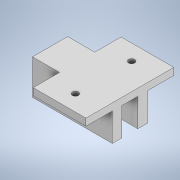
# Autodesk Inventor part: pulleysupport
Saved by Autodesk Inventor 2020.2 (Build 242310000, 310)
## iProperties
Created: 2020-08-06
Part Number: pulleysupport
Material: Generic
Document SubType Name: Modeling
Designer: JK
Density: 1 g/cm^3
Appearance: Default
Author: JK
Autodesk Inventor part; units mm, degrees
ref_plane "YZ Plane" through (0, 0, 0) normal (1, 0, 0) x (0, 1, 0)
ref_plane "XZ Plane" through (0, 0, 0) normal (0, 1, 0) x (-1, 0, 0)
ref_plane "XY Plane" through (0, 0, 0) normal (0, 0, 1) x (1, 0, 0)
sketch "Sketch1" plane through (0, 0, 0) normal (0, 1, 0) x (-1, 0, 0)
  line L0 (-15, 25) -> (15, 25)
  line L1 (15, 25) -> (15, -25)
  line L2 (15, -25) -> (-15, -25)
  line L3 (-15, -25) -> (-15, 25)
  line L4 (-15, 25) -> (15, -25) construction
  line L5 (15, 25) -> (-15, -25) construction
  circle A0 centre (0, 16) radius 1.75
  circle A1 centre (0, -16) radius 1.75
  point P0 (0, 0)
  dimension "d0" = 3.5
  dimension "d1" = 30
  dimension "d2" = 50
  dimension "d3" = 16
  dimension "d4" = 16
  constraints: 12 end point, 2 centre point, 2 midpoint, 2 parallel, 1 equal radius, 1 horizontal, 1 perpendicular
  measures "d0" diameter of A0
  measures "d1" distance of L0.start L0.end
  measures "d2" distance of L0.end L1.end
  measures "d3" distance of A0.centre point (0, 0)
  measures "d4" distance of A1.centre point (0, 0)
extrude "Extrusion1" add sketch "Sketch1" along normal blind 4
sketch "Sketch2" plane through (0, 4, 0) normal (0, 1, 0) x (1, 0, 0)
  line L0 (15, -25) -> (15, 25) projected
  line L1 (15, -10) -> (-30.3844, -10)
  line L2 (-30.3844, -10) -> (-30.3844, 10)
  line L3 (-30.3844, 10) -> (15, 10)
  line L4 (15, 10) -> (15, -10)
  line L5 (-15, -25) -> (15, -25) projected
  point P0 (0, 0)
  point P1 (15, 10)
  dimension "d9" = 20
  dimension "d11" = 10
  constraints: 8 end point, 2 parallel, 1 horizontal, 1 perpendicular, 1 point on line
  measures "d9" distance between parallel lines of L1 L3
  measures "d11" distance from line of L1 point (0, 0)
extrude "Extrusion2" add sketch "Sketch2" against normal blind 20
sketch "Sketch3" plane through (0, -16, 0) normal (0, -1, 0) x (1, 0, 0)
  point P0 (0, 0)
sketch "Sketch4" plane through (0, -16, 0) normal (0, -1, 0) x (1, 0, 0)
  line L0 (33.9353, -4.5) -> (-33.9353, -4.5)
  line L1 (-33.9353, -4.5) -> (-33.9353, 4.5)
  line L2 (-33.9353, 4.5) -> (33.9353, 4.5)
  line L3 (33.9353, 4.5) -> (33.9353, -4.5)
  line L4 (33.9353, -4.5) -> (-33.9353, 4.5) construction
  line L5 (-33.9353, -4.5) -> (33.9353, 4.5) construction
  point P0 (0, 0)
  dimension "d12" = 9
  constraints: 12 end point, 2 midpoint, 2 parallel, 1 horizontal, 1 perpendicular
  measures "d12" distance between parallel lines of L2 L0
extrude "Extrusion3" cut sketch "Sketch4" against normal up to surface (16 mm away)
body "Solid1"
